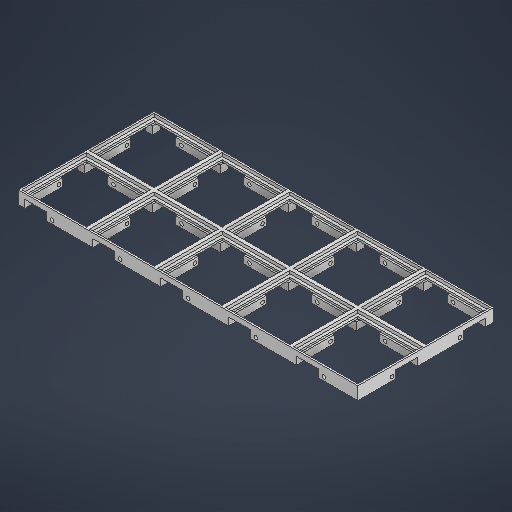
# Autodesk Inventor part: PCB_holder_field_5x2
Saved by Autodesk Inventor 2026.2 (Build 302298010, 298A)
## iProperties
Created: 2026-03-12
Part Number: PCB_holder_field_5x2
Material: Generisch
Document SubType Name: Modeling
Designer: ami-student
Density: 1 g/cm^3
Appearance: Vorgabe
Author: ami-student
Autodesk Inventor part; units mm, degrees
note: some values were not read from the file. Chosen so that the rebuilt part matches the saved one: direction of "Bohrung2".
ref_plane "YZ Plane" through (0, 0, 0) normal (1, 0, 0) x (0, 1, 0)
ref_plane "XZ Plane" through (0, 0, 0) normal (0, 1, 0) x (-1, 0, 0)
ref_plane "XY Plane" through (0, 0, 0) normal (0, 0, 1) x (1, 0, 0)
sketch "Skizze1" plane through (0, 0, 0) normal (0, 0, 1) x (1, 0, 0)
  line L0 (-28.13, 28.13) -> (28.13, 28.13)
  line L1 (28.13, 28.13) -> (28.13, -28.13)
  line L2 (28.13, -28.13) -> (-28.13, -28.13)
  line L3 (-28.13, -28.13) -> (-28.13, 28.13)
  line L4 (0, -39.382) -> (0, 39.382) construction
  line L5 (-39.382, 0) -> (39.382, 0) construction
  point P0 (0, 0)
  dimension "d0" = 56.26
  constraints: 8 end point, 2 parallel, 2 perpendicular, 1 horizontal, 2 other
  measures "d0" distance of L2.end L0.start
extrude "Extrusion1" add sketch "Skizze1" along normal blind 10.6
sketch "Skizze2" plane through (0, 0, 10.6) normal (0, 0, 1) x (1, 0, 0)
  line L0 (-39.382, 0) -> (39.382, 0) construction
  line L1 (0, -39.382) -> (0, 39.382) construction
  line L2 (-26.655, 26.655) -> (26.655, 26.655)
  line L3 (26.655, 26.655) -> (26.655, -26.655)
  line L4 (26.655, -26.655) -> (-26.655, -26.655)
  line L5 (-26.655, -26.655) -> (-26.655, 26.655)
  point P0 (0, 0)
  dimension "d3" = 53.31
  constraints: 8 end point, 2 parallel, 2 perpendicular, 1 horizontal, 2 other
  measures "d3" distance of L4.end L2.start
extrude "Extrusion2" cut sketch "Skizze2" against normal blind 2.6
sketch "Skizze3" plane through (0, 0, 8) normal (0, 0, 1) x (1, 0, 0)
  line L0 (-24.18, 24.18) -> (24.18, 24.18)
  line L1 (24.18, 24.18) -> (24.18, -24.18)
  line L2 (24.18, -24.18) -> (-24.18, -24.18)
  line L3 (-24.18, -24.18) -> (-24.18, 24.18)
  line L4 (-39.382, 0) -> (39.382, 0) construction
  line L5 (0, -39.382) -> (0, 39.382) construction
  line L6 (-26.655, -26.655) -> (-26.655, 26.655) projected
  point P0 (0, 0)
  dimension "d7" = 2.475
  constraints: 8 end point, 2 parallel, 2 perpendicular, 1 horizontal, 2 other
  measures "d7" distance between parallel lines of L6 L3
extrude "Extrusion3" cut sketch "Skizze3" against normal blind 1.6
sketch "Skizze4" plane through (0, 0, 6.4) normal (0, 0, 1) x (1, 0, 0)
  line L0 (0, -39.382) -> (0, 39.382) construction
  line L1 (-39.382, 0) -> (39.382, 0) construction
  line L2 (-22.63, 22.63) -> (22.63, 22.63)
  line L3 (22.63, 22.63) -> (22.63, -22.63)
  line L4 (22.63, -22.63) -> (-22.63, -22.63)
  line L5 (-22.63, -22.63) -> (-22.63, 22.63)
  point P0 (0, 0)
  dimension "d10" = 45.26
  constraints: 8 end point, 2 parallel, 2 perpendicular, 1 horizontal, 2 other
  measures "d10" distance of L4.end L2.start
extrude "Extrusion4" cut sketch "Skizze4" against normal up to surface (6.4 mm away)
sketch "Skizze5" plane through (-28.13, -28.13, 0) normal (-1, 0, 0) x (0, 0, 1)
  line L0 (0, 49.26) -> (6.4, 49.26)
  line L1 (6.4, 49.26) -> (6.4, 31.26)
  line L2 (6.4, 31.26) -> (0, 31.26)
  line L3 (0, 31.26) -> (0, 49.26)
  line L4 (0, 56.26) -> (0, 0) projected
  line L5 (0, 0) -> (10.6, 0) projected
  line L6 (10.6, 56.26) -> (10.6, 0) projected
  line L7 (0, 56.26) -> (10.6, 56.26) projected
  point P0 (0, 28.13)
  point P1 (3.2, 49.26)
  dimension "d13" = 7
  dimension "d14" = 18
  dimension "d15" = 6.4
  constraints: 8 end point, 2 parallel, 1 collinear, 1 horizontal, 1 midpoint, 1 perpendicular
  measures "d13" distance between parallel lines of L7 L0
  measures "d14" distance from line of L2 point (3.2, 49.26)
  measures "d15" distance of L0.start L0.end
extrude "Extrusion5" cut sketch "Skizze5" against normal up to surface (56.26 mm away) contours L0 L1 L2 L3
sketch "Skizze6" plane through (-28.13, 28.13, 0) normal (0, 1, 0) x (1, 0, 0)
  line L0 (5.5, 0) -> (0, 0) projected
  line L1 (5.5, 0) -> (23.5, 0)
  line L2 (23.5, 0) -> (23.5, -6.4)
  line L3 (23.5, -6.4) -> (5.5, -6.4)
  line L4 (5.5, -6.4) -> (5.5, 0)
  point P0 (28.13, 0)
  dimension "d18" = 18
  dimension "d19" = 6.4
  constraints: 8 end point, 2 parallel, 1 horizontal, 1 perpendicular
  measures "d18" distance between parallel lines of L2 L4
  measures "d19" distance of L3.end L0.start
extrude "Extrusion6" cut sketch "Skizze6" against normal up to surface (56.26 mm away)
sketch "Skizze7" plane through (0, 0, 0) normal (0, 0, -1) x (-1, 0, 0)
  line L0 (28.13, 28.13) -> (28.13, 21.13) projected
  line L1 (-28.13, 28.13) -> (4.63, 28.13) projected
  point P0 (0, 0)
  point P1 (5, 25.38)
  point P2 (-5, 25.38)
  dimension "d22" = 23.13
  dimension "d23" = 33.13
  dimension "d24" = 2.75
  dimension "d25" = 2.75
  measures "d22" distance from line of L0 point (5, 25.38)
  measures "d23" distance from line of point (-5, 25.38) L0
  measures "d24" distance from line of L1 point (-5, 25.38)
  measures "d25" distance from line of L1 point (5, 25.38)
hole "Bohrung1" [suppressed]
sketch "Skizze8" plane through (22.63, 22.63, 0) normal (0, -1, 0) x (1, 0, 0)
  line L0 (0, 0) -> (-27.26, 0) projected
  line L1 (-50.76, 0) -> (-50.76, 10.6) projected
  point P0 (-22.63, 0)
  point P1 (-22.63, 3)
  dimension "d33" = 3
  dimension "d42" = 28.13
  measures "d33" distance from line of L0 point (-22.63, 3)
  measures "d42" distance from line of L1 point (-22.63, 3)
hole "Bohrung2" at (0, 22.63, 3) direction (0, 1, 0) diameter 3 depth 5.5
pattern_circular "Runde Anordnung1" count 4 over 360 about axis through (0, 0, -10) along (0, 0, 1) of "Bohrung2"
pattern_linear "Rechteckige Anordnung1" count 5 spacing 56.26 along (1, 0, 0) count 2 spacing 56.26 along (0, 1, 0) of "Extrusion1", "Extrusion2", "Extrusion3", "Extrusion4", "Extrusion5", "Extrusion6", "Bohrung2", "Runde Anordnung1"
